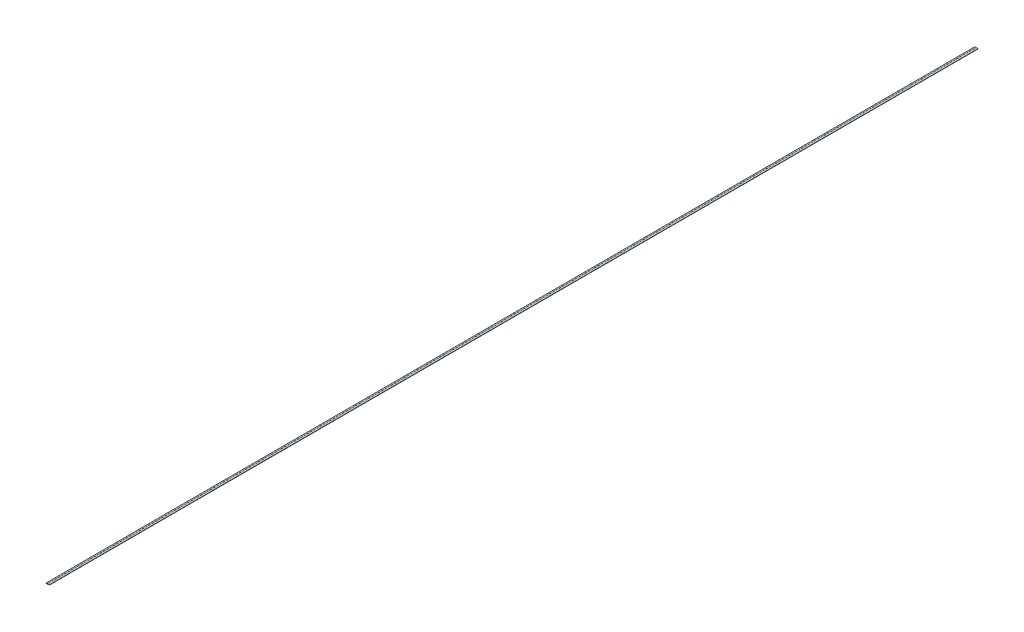
# Autodesk Inventor part: SP40-14 PERFIL RETICULAR TRAVESAÑO
Saved by Autodesk Inventor 2025 (Build 290162000, 162)
## iProperties
Created: 2026-01-30
Part Number: SP40-14 PERFIL RETICULAR TRAVESAÑO
Material: Aluminio
Document SubType Name: Modeling
Designer: ROLANDO
Density: 2.7 g/cm^3
Appearance: Satinado
Author: ROLANDO
Autodesk Inventor part; units mm, degrees
ref_plane "YZ Plane" through (0, 0, 0) normal (1, 0, 0) x (0, 1, 0)
ref_plane "XZ Plane" through (0, 0, 0) normal (0, 1, 0) x (-1, 0, 0)
ref_plane "XY Plane" through (0, 0, 0) normal (0, 0, 1) x (1, 0, 0)
sketch "Boceto1" plane through (0, 0, 0) normal (0, 0, 1) x (1, 0, 0)
  line L0 (0, -2.926) -> (0, 4.2457) construction
  line L1 (-0.5, 1.2) -> (-0.5, 1.2888)
  line L2 (-0.7, 1) -> (-1.3, 1)
  line L3 (-1.5, 0.8) -> (-1.5, 0.2)
  line L4 (-9, 0) -> (-8, 0)
  line L5 (-8, 0) -> (-8, 0.0947)
  line L6 (-9, 0) -> (-9, 0.9017)
  arc A0 (-0.3, 2.5112) -> (-8.6098, 1.3895) centre (1.9614, -45.5856) ccw
  arc A1 (-0.7113, 1.4885) -> (-7.6014, 0.5844) centre (1.9614, -45.5856) ccw
  line L7 (0.5, 1.2) -> (0.5, 1.2888)
  line L8 (0.7, 1) -> (1.3, 1)
  line L9 (1.5, 0.8) -> (1.5, 0.2)
  line L10 (9, 0) -> (8, 0)
  line L11 (8, 0) -> (8, 0.0947)
  line L12 (9, 0) -> (9, 0.9017)
  arc A2 (8.6098, 1.3895) -> (0.3, 2.5112) centre (-1.9614, -45.5856) ccw
  arc A3 (7.6014, 0.5844) -> (0.7113, 1.4885) centre (-1.9614, -45.5856) ccw
  line L13 (1.3, 0) -> (-1.3, 0)
  arc A4 (-0.3, 2.5112) -> (0.3, 2.5112) centre (0, 2.5112) ccw
  arc A5 (-8.6098, 1.3895) -> (-9, 0.9017) centre (-8.5, 0.9017) ccw
  arc A6 (-7.6014, 0.5844) -> (-8, 0.0947) centre (-7.5, 0.0947) ccw
  arc A7 (8, 0.0947) -> (7.6014, 0.5844) centre (7.5, 0.0947) ccw
  arc A8 (9, 0.9017) -> (8.6098, 1.3895) centre (8.5, 0.9017) ccw
  arc A9 (-0.7, 1) -> (-0.5, 1.2) centre (-0.7, 1.2) ccw
  arc A10 (-0.5, 1.2888) -> (-0.7113, 1.4885) centre (-0.7, 1.2888) ccw
  arc A11 (0.7113, 1.4885) -> (0.5, 1.2888) centre (0.7, 1.2888) ccw
  arc A12 (0.5, 1.2) -> (0.7, 1) centre (0.7, 1.2) ccw
  arc A13 (1.5, 0.8) -> (1.3, 1) centre (1.3, 0.8) ccw
  arc A14 (1.3, 0) -> (1.5, 0.2) centre (1.3, 0.2) ccw
  arc A15 (-1.5, 0.2) -> (-1.3, 0) centre (-1.3, 0.2) ccw
  arc A16 (-1.3, 1) -> (-1.5, 0.8) centre (-1.3, 0.8) ccw
  line L14 (-1.0156, 2.5112) -> (0.9053, 2.5112) construction
  point P0 (0, 0)
  point P1 (-0.5, 1)
  point P2 (-1.5, 1)
  point P3 (-1.5, 0)
  point P4 (-8, 0.5)
  point P5 (-9, 1.3)
  point P6 (-0.5, 1.5)
  point P7 (8, 0.5)
  point P8 (9, 1.3)
  point P9 (0.5, 1.5)
  dimension "d21" = 1
  dimension "d26" = 0.5
  dimension "d31" = 1
  dimension "d34" = 0.5
  dimension "d35" = 1.3
  dimension "d37" = 1
  dimension "d38" = 0.5
  dimension "d39" = 9
  dimension "d41" = 1
  dimension "d42" = 3
  dimension "d43" = 1.5
  dimension "d44" = 1.5
  dimension "d45" = 1
  dimension "d46" = 1.3
  dimension "d47" = 0.5
  dimension "d48" = 1
  dimension "d49" = 18
  dimension "d56" = 0.6
  dimension "d63" = 0.5
  dimension "d64" = 0.2
  dimension "d66" = 2.5112
  constraints: 40 point on circle, 30 end point, 24 tangent, 17 centre point, 15 point on line, 11 equal radius, 5 horizontal, 4 vertical, 3 collinear, 2 coincident, 2 perpendicular, 1 midpoint, 1 parallel
  measures "d21" distance of L4.start L4.end
  measures "d26" distance of L4.end point (-8, 0.5)
  measures "d31" radial gap between concentric circles of A0 A1
  measures "d34" distance of point (-0.5, 1) point (-0.5, 1.5)
  measures "d35" distance of L4.start point (-9, 1.3)
  measures "d37" distance of point (-1.5, 1) point (-1.5, 0)
  measures "d38" distance between parallel lines of L0 L1
  measures "d39" distance between parallel lines of L0 L6
  measures "d41" distance of L10.start L10.end
  measures "d42" distance between parallel lines of L9 L3
  measures "d43" distance between parallel lines of L0 L9
  measures "d44" distance between parallel lines of L0 L3
  measures "d45" distance between parallel lines of L1 L7
  measures "d46" distance of L10.start point (9, 1.3)
  measures "d47" distance of L10.end point (8, 0.5)
  measures "d48" radial gap between concentric circles of A2 A3
  measures "d49" distance between parallel lines of L6 L12
  measures "d56" diameter of A4
  measures "d63" radius of A5
  measures "d64" radius of A9
  measures "d66" distance from line of L13 A4.centre
extrude "Extrusión1" add sketch "Boceto1" against normal blind 5000
